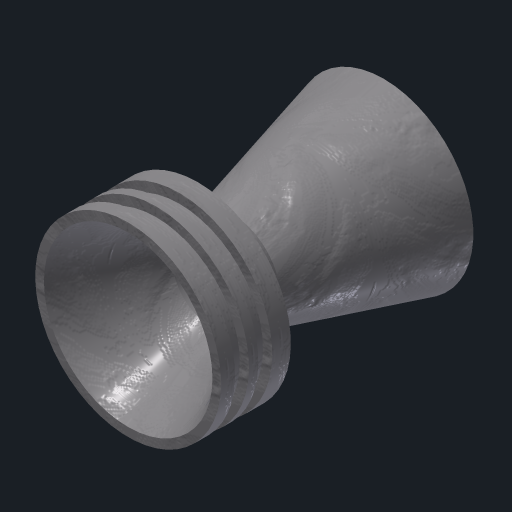
# Autodesk Inventor part: TOBERA
Saved by Autodesk Inventor 2024.3 (Build 283343000, 343)
## iProperties
Created: 2024-08-15
Part Number: TOBERA
Material: Steel, Mild, Welded
Document SubType Name: Modeling
Designer: Niler
Density: 7.85 g/cm^3
Appearance: Weld - Steel Mild
Author: Niler
Autodesk Inventor part; units mm, degrees
ref_plane "YZ Plane" through (0, 0, 0) normal (1, 0, 0) x (0, 1, 0)
ref_plane "XZ Plane" through (0, 0, 0) normal (0, 1, 0) x (-1, 0, 0)
ref_plane "XY Plane" through (0, 0, 0) normal (0, 0, 1) x (1, 0, 0)
sketch "Sketch1" plane through (0, 0, 0) normal (1, 0, 0) x (0, 1, 0)
  line L0 (0, 0) -> (20, 0)
  line L1 (20, 0) -> (20, -15)
  line L2 (20, -15) -> (13, -15)
  line L3 (13, -15) -> (10.5, -22.3073)
  line L4 (10.5, -22.3073) -> (19.26, -55)
  line L5 (19.26, -55) -> (0, -55)
  line L6 (0, 0) -> (0, -55)
  line L7 (17.5, -55) -> (8, -19.5455)
  line L8 (8, -19.5455) -> (8, -17.5455)
  line L9 (8, -17.5455) -> (18.1299, 0)
  line L10 (20, -3) -> (18, -3)
  line L11 (18, -3) -> (18, -6)
  line L12 (18, -6) -> (20, -6)
  line L13 (20, -6) -> (20, -3)
  line L14 (20, -8) -> (18, -8)
  line L15 (18, -8) -> (18, -11)
  line L16 (18, -11) -> (20, -11)
  line L17 (20, -11) -> (20, -8)
  dimension "d0" = 1.7
  dimension "d1" = 55
  dimension "d2" = 15
  dimension "d3" = 15
  dimension "d4" = 30
  dimension "d5" = 8
  dimension "d6" = 20
  dimension "d7" = 17.5
  dimension "d8" = 2
  dimension "d9" = 13
  dimension "d10" = 10.5
  dimension "d11" = 2
  dimension "d12" = 3
  dimension "d13" = 3
  dimension "d14" = 8
  constraints: 36 end point, 5 parallel, 4 perpendicular, 4 point on line, 3 horizontal, 2 equal length, 1 vertical, 1 vertical alignment
  measures "d0" distance between parallel lines of L7 L4
  measures "d1" distance between parallel lines of L5 L0
  measures "d2" distance between parallel lines of L0 L2
  measures "d3" angle of L6 L7
  measures "d4" angle of L6 L9
  measures "d5" distance between parallel lines of L6 L8
  measures "d6" distance between parallel lines of L6 L1
  measures "d7" distance of L5.end L7.start
  measures "d8" distance of L7.end L8.end
  measures "d9" distance from line of L6 L2.end
  measures "d10" distance from line of L6 L3.end
  measures "d11" distance of L11.end L12.end
  measures "d12" distance of L12.end L10.start
  measures "d13" distance between parallel lines of L0 L10
  measures "d14" distance between parallel lines of L0 L14
revolve "Revolution1" add sketch "Sketch1" angle 360 about axis through (0, 0, 0) along (0, 0, -1) contours L0 L1 L10 L11 L12 L14 L15 L16 L2 L3 L4 L5 L7 L8 L9
body "Solid1"
